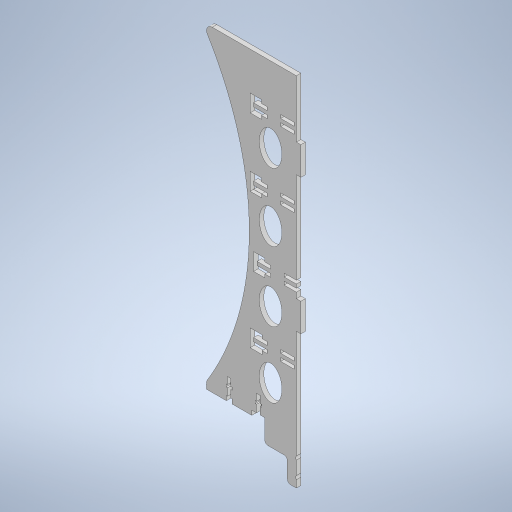
# Autodesk Inventor part: ребро0.5
Saved by Autodesk Inventor 2023.1 (Build 271208000, 208)
## iProperties
Created: 2025-01-17
Part Number: ребро0.5
Material: Типовые
Document SubType Name: Modeling
Designer: Коноваленко
Density: 1 g/cm^3
Appearance: По умолчанию
Author: Коноваленко
Autodesk Inventor part; units mm, degrees
(part 1 of 2)
ref_plane "YZ Plane" through (0, 0, 0) normal (1, 0, 0) x (0, 1, 0)
ref_plane "XZ Plane" through (0, 0, 0) normal (0, 1, 0) x (-1, 0, 0)
ref_plane "XY Plane" through (0, 0, 0) normal (0, 0, 1) x (1, 0, 0)
sketch "Эскиз1" plane through (0, 0, 0) normal (0, 0, 1) x (1, 0, 0)
  line L0 (81.8324, 0) -> (81.8324, -4) construction
  line L1 (72.759, -4) -> (11.9953, -4)
  line L2 (11.9953, -4) -> (11.9953, 0) construction
  line L3 (11.9953, 0) -> (81.8324, 0) construction
  line L4 (-75.5314, 0) -> (7.9958, 0) construction
  line L5 (7.9958, 0) -> (7.9958, -4) construction
  line L6 (7.9958, -4) -> (-66.4579, -4)
  line L7 (-75.5314, -4) -> (-75.5314, 0) construction
  line L8 (7.9953, 276) -> (11.9953, 276) construction
  line L9 (-75.5314, 0) -> (81.8324, 0)
  line L10 (72.759, 276) -> (-66.4579, 276)
  arc A0 (-70.7311, 3.5962) -> (-70.7311, 268.4038) centre (-288.6628, 136) ccw
  line L11 (3.1505, 276) -> (3.1505, 0) construction
  arc A1 (77.0322, 268.4038) -> (77.0322, 3.5962) centre (294.9639, 136) ccw
  arc A2 (-66.4579, 276) -> (-70.7311, 268.4038) centre (-66.4579, 271) ccw
  arc A3 (77.0322, 268.4038) -> (72.759, 276) centre (72.759, 271) ccw
  arc A4 (-70.7311, 3.5962) -> (-66.4579, -4) centre (-66.4579, 1) ccw
  arc A5 (72.759, -4) -> (77.0322, 3.5962) centre (72.759, 1) ccw
  point P0 (81.8324, 276)
  point P1 (-75.5314, 276)
  point P2 (-71.3569, 0)
  point P3 (77.658, 0)
  dimension "d0" = 255
  dimension "d1" = 5
  constraints: 24 end point, 16 point on circle, 8 tangent, 6 centre point, 4 point on line, 3 equal radius, 2 midpoint, 1 horizontal, 1 parallel, 1 symmetric about line, 1 other
  measures "d0" radius of A0
  measures "d1" radius of A2
extrude "Выдавливание1" add sketch "Эскиз1" along normal blind 4
sketch "Эскиз2" plane through (0, 0, 4) normal (0, 0, 1) x (1, 0, 0)
  line L0 (-29.8867, 53.1563) -> (-17.8867, 53.1563)
  line L1 (42.1133, 53.1563) -> (42.1133, 54.9927) construction
  line L2 (-29.8867, 50.1563) -> (-29.8867, 53.1563)
  line L3 (6.1133, 50.1563) -> (6.1133, 53.1563)
  line L4 (6.1133, 50.1563) -> (6.1133, 53.1563) construction
  line L5 (-17.8867, 50.1563) -> (-17.8867, 53.1563)
  line L6 (-5.8867, 50.1563) -> (-5.8867, 53.1563)
  line L7 (18.1133, 50.1563) -> (18.1133, 53.1563)
  line L8 (30.1133, 50.1563) -> (30.1133, 53.1563)
  line L9 (-17.8867, 50.1563) -> (-29.8867, 50.1563)
  line L10 (-17.8867, 53.1563) -> (-5.8867, 53.1563) construction
  line L11 (-5.8867, 53.1563) -> (6.1133, 53.1563)
  line L12 (-5.8867, 50.1563) -> (-17.8867, 50.1563) construction
  line L13 (6.1133, 53.1563) -> (18.1133, 53.1563) construction
  line L14 (18.1133, 50.1563) -> (6.1133, 50.1563) construction
  line L15 (18.1133, 53.1563) -> (30.1133, 53.1563)
  line L16 (30.1133, 53.1563) -> (42.1133, 53.1563) construction
  line L17 (30.1133, 50.1563) -> (18.1133, 50.1563)
  line L18 (6.1133, 50.1563) -> (-5.8867, 50.1563)
  line L19 (6.1133, 6.0367) -> (6.1133, 56.3563) construction
  line L20 (-29.8867, 59.3563) -> (-17.8867, 59.3563)
  line L21 (42.1133, 59.3563) -> (42.1133, 56.3563) construction
  line L22 (42.1133, 56.3563) -> (30.1133, 56.3563) construction
  line L23 (-29.8867, 56.3563) -> (-29.8867, 59.3563)
  line L24 (6.1133, 56.3563) -> (6.1133, 59.3563)
  line L25 (6.1133, 56.3563) -> (6.1133, 59.3563) construction
  line L26 (-17.8867, 56.3563) -> (-17.8867, 59.3563)
  line L27 (-5.8867, 56.3563) -> (-5.8867, 59.3563)
  line L28 (18.1133, 56.3563) -> (18.1133, 59.3563)
  line L29 (30.1133, 56.3563) -> (30.1133, 59.3563)
  line L30 (-17.8867, 56.3563) -> (-29.8867, 56.3563)
  line L31 (-17.8867, 59.3563) -> (-5.8867, 59.3563) construction
  line L32 (-5.8867, 59.3563) -> (6.1133, 59.3563)
  line L33 (-5.8867, 56.3563) -> (-17.8867, 56.3563) construction
  line L34 (6.1133, 59.3563) -> (18.1133, 59.3563) construction
  line L35 (18.1133, 56.3563) -> (6.1133, 56.3563) construction
  line L36 (18.1133, 59.3563) -> (30.1133, 59.3563)
  line L37 (30.1133, 59.3563) -> (42.1133, 59.3563) construction
  line L38 (30.1133, 56.3563) -> (18.1133, 56.3563)
  line L39 (6.1133, 56.3563) -> (-5.8867, 56.3563)
  line L40 (6.1133, -16.2034) -> (6.1133, 259.7966) construction
  line L41 (72.759, 276) -> (-66.4579, 276) projected
  line L42 (9.2728, 110.1563) -> (9.2728, 113.1563)
  line L43 (9.2728, 110.1563) -> (9.2728, 113.1563) construction
  line L44 (-2.8167, 113.1563) -> (9.2728, 113.1563)
  line L45 (9.2728, 110.1563) -> (-2.8167, 110.1563)
  line L46 (-2.8167, 110.1563) -> (-2.8167, 113.1563)
  line L47 (-14.8167, 110.1563) -> (-14.8167, 113.1563)
  line L48 (-14.8167, 113.1563) -> (-2.8167, 113.1563) construction
  line L49 (-2.8167, 110.1563) -> (-14.8167, 110.1563) construction
  line L50 (9.2728, 55.0001) -> (9.2728, 110.1563) construction
  line L51 (21.2728, 110.1563) -> (9.2728, 110.1563) construction
  line L52 (9.2728, 113.1563) -> (21.2728, 113.1563) construction
  line L53 (21.2728, 110.1563) -> (21.2728, 113.1563)
  line L54 (33.2728, 110.1563) -> (21.2728, 110.1563)
  line L55 (21.2728, 113.1563) -> (33.2728, 113.1563)
  line L56 (33.2728, 110.1563) -> (33.2728, 113.1563)
  line L57 (45.1508, 113.1563) -> (45.1508, 110.1563) construction
  line L58 (33.2728, 113.1563) -> (45.1508, 113.1563) construction
  line L59 (-26.8167, 113.1563) -> (-14.8167, 113.1563)
  line L60 (-26.8167, 110.1563) -> (-26.8167, 113.1563)
  line L61 (-14.8167, 110.1563) -> (-26.8167, 110.1563)
  line L62 (-14.8167, 116.3563) -> (-14.8167, 119.3563)
  line L63 (-26.8167, 119.3563) -> (-14.8167, 119.3563)
  line L64 (-14.8167, 116.3563) -> (-26.8167, 116.3563)
  line L65 (21.2728, 116.3563) -> (21.2728, 119.3563)
  line L66 (21.2728, 119.3563) -> (33.2728, 119.3563)
  line L67 (33.2728, 116.3563) -> (33.2728, 119.3563)
  line L68 (33.2728, 116.3563) -> (21.2728, 116.3563)
  line L69 (45.1833, 119.3563) -> (45.1833, 116.3563) construction
  line L70 (21.2728, 116.3563) -> (9.2728, 116.3563) construction
  line L71 (9.2728, 119.3563) -> (21.2728, 119.3563) construction
  line L72 (9.2728, 116.3563) -> (9.2728, 119.3563)
  line L73 (9.2728, 116.3563) -> (9.2728, 119.3563) construction
  line L74 (-26.8167, 116.3563) -> (-26.8167, 119.3563)
  line L75 (33.2728, 119.3563) -> (45.1833, 119.3563) construction
  line L76 (-14.8167, 119.3563) -> (-2.8167, 119.3563) construction
  line L77 (-2.8167, 116.3563) -> (-2.8167, 119.3563)
  line L78 (-2.8167, 119.3563) -> (9.2728, 119.3563)
  line L79 (9.2728, 116.3563) -> (-2.8167, 116.3563)
  line L80 (-2.8167, 116.3563) -> (-14.8167, 116.3563) construction
  line L81 (45.1833, 116.3563) -> (33.2728, 116.3563) construction
  line L82 (6.1133, 170.1563) -> (6.1133, 173.1563)
  line L83 (6.1133, 170.1563) -> (6.1133, 173.1563) construction
  line L84 (-5.8867, 173.1563) -> (6.1133, 173.1563)
  line L85 (6.1133, 170.1563) -> (-5.8867, 170.1563)
  line L86 (-5.8867, 170.1563) -> (-5.8867, 173.1563)
  line L87 (-17.8867, 170.1563) -> (-17.8867, 173.1563)
  line L88 (-17.8867, 173.1563) -> (-5.8867, 173.1563) construction
  line L89 (-5.8867, 170.1563) -> (-17.8867, 170.1563) construction
  line L90 (18.1133, 170.1563) -> (6.1133, 170.1563) construction
  line L91 (6.1133, 173.1563) -> (18.1133, 173.1563) construction
  line L92 (18.1133, 170.1563) -> (18.1133, 173.1563)
  line L93 (30.1133, 170.1563) -> (18.1133, 170.1563)
  line L94 (18.1133, 173.1563) -> (30.1133, 173.1563)
  line L95 (30.1133, 170.1563) -> (30.1133, 173.1563)
  line L96 (42.1133, 170.1563) -> (30.1133, 170.1563) construction
  line L97 (42.1133, 173.1563) -> (42.1133, 170.1563) construction
  line L98 (30.1133, 173.1563) -> (42.1133, 173.1563) construction
  line L99 (-29.8867, 173.1563) -> (-17.8867, 173.1563)
  line L100 (-29.8867, 170.1563) -> (-29.8867, 173.1563)
  line L101 (-17.8867, 170.1563) -> (-29.8867, 170.1563)
  line L102 (6.1133, 179.3563) -> (18.1133, 179.3563) construction
  line L103 (18.1133, 176.3563) -> (6.1133, 176.3563) construction
  line L104 (18.1133, 176.3563) -> (18.1133, 179.3563)
  line L105 (30.1133, 176.3563) -> (18.1133, 176.3563)
  line L106 (18.1133, 179.3563) -> (30.1133, 179.3563)
  line L107 (-29.8867, 179.3563) -> (-17.8867, 179.3563)
  line L108 (-17.8867, 176.3563) -> (-29.8867, 176.3563)
  line L109 (-29.8867, 176.3563) -> (-29.8867, 179.3563)
  line L110 (-17.8867, 176.3563) -> (-17.8867, 179.3563)
  line L111 (30.1133, 176.3563) -> (30.1133, 179.3563)
  line L112 (42.1133, 176.3563) -> (30.1133, 176.3563) construction
  line L113 (42.1133, 179.3563) -> (42.1133, 176.3563) construction
  line L114 (30.1133, 179.3563) -> (42.1133, 179.3563) construction
  line L115 (-5.8867, 176.3563) -> (-17.8867, 176.3563) construction
  line L116 (-17.8867, 179.3563) -> (-5.8867, 179.3563) construction
  line L117 (-5.8867, 176.3563) -> (-5.8867, 179.3563)
  line L118 (6.1133, 176.3563) -> (-5.8867, 176.3563)
  line L119 (-5.8867, 179.3563) -> (6.1133, 179.3563)
  line L120 (6.1133, 176.3563) -> (6.1133, 179.3563)
  line L121 (6.1133, 176.3563) -> (6.1133, 179.3563) construction
  line L122 (6.1133, 233.1563) -> (18.1133, 233.1563) construction
  line L123 (18.1133, 230.1563) -> (6.1133, 230.1563) construction
  line L124 (18.1133, 230.1563) -> (18.1133, 233.1563)
  line L125 (30.1133, 230.1563) -> (18.1133, 230.1563)
  line L126 (18.1133, 233.1563) -> (30.1133, 233.1563)
  line L127 (-29.8867, 233.1563) -> (-17.8867, 233.1563)
  line L128 (-17.8867, 230.1563) -> (-29.8867, 230.1563)
  line L129 (-29.8867, 230.1563) -> (-29.8867, 233.1563)
  line L130 (-17.8867, 230.1563) -> (-17.8867, 233.1563)
  line L131 (30.1133, 230.1563) -> (30.1133, 233.1563)
  line L132 (42.1133, 230.1563) -> (30.1133, 230.1563) construction
  line L133 (42.1133, 233.1563) -> (42.1133, 230.1563) construction
  line L134 (30.1133, 233.1563) -> (42.1133, 233.1563) construction
  line L135 (-5.8867, 230.1563) -> (-17.8867, 230.1563) construction
  line L136 (-17.8867, 233.1563) -> (-5.8867, 233.1563) construction
  line L137 (-5.8867, 230.1563) -> (-5.8867, 233.1563)
  line L138 (6.1133, 230.1563) -> (-5.8867, 230.1563)
  line L139 (-5.8867, 233.1563) -> (6.1133, 233.1563)
  line L140 (6.1133, 230.1563) -> (6.1133, 233.1563)
  line L141 (6.1133, 230.1563) -> (6.1133, 233.1563) construction
  line L142 (18.1133, 236.3563) -> (18.1133, 239.3563)
  line L143 (30.1133, 236.3563) -> (18.1133, 236.3563)
  line L144 (18.1133, 239.3563) -> (30.1133, 239.3563)
  line L145 (30.1133, 236.3563) -> (30.1133, 239.3563)
  line L146 (42.1133, 236.3563) -> (30.1133, 236.3563) construction
  line L147 (30.1133, 239.3563) -> (42.1133, 239.3563) construction
  line L148 (42.1133, 239.3563) -> (42.1133, 236.3563) construction
  line L149 (18.1133, 236.3563) -> (6.1133, 236.3563) construction
  line L150 (6.1133, 239.3563) -> (18.1133, 239.3563) construction
  line L151 (6.1133, 236.3563) -> (6.1133, 239.3563)
  line L152 (6.1133, 236.3563) -> (6.1133, 239.3563) construction
  line L153 (6.1133, 236.3563) -> (-5.8867, 236.3563)
  line L154 (-5.8867, 239.3563) -> (6.1133, 239.3563)
  line L155 (-5.8867, 236.3563) -> (-5.8867, 239.3563)
  line L156 (-5.8867, 236.3563) -> (-17.8867, 236.3563) construction
  line L157 (-17.8867, 239.3563) -> (-5.8867, 239.3563) construction
  line L158 (-17.8867, 236.3563) -> (-17.8867, 239.3563)
  line L159 (-29.8867, 239.3563) -> (-17.8867, 239.3563)
  line L160 (-29.8867, 236.3563) -> (-29.8867, 239.3563)
  line L161 (-17.8867, 236.3563) -> (-29.8867, 236.3563)
  arc A0 (-70.7311, 3.5962) -> (-70.7311, 268.4038) centre (-288.6628, 136) ccw construction
  arc A1 (77.0322, 268.4038) -> (77.0322, 3.5962) centre (294.9639, 136) ccw construction
  line L162 (11.994, 50.1563) -> (7.994, 50.1563) projected
  line L163 (11.994, 110.1563) -> (7.994, 110.1563) projected
  line L164 (11.9939, 170.1563) -> (7.9939, 170.1563) projected
  line L165 (11.9939, 230.1563) -> (7.9939, 230.1563) projected
  point P0 (0, 0)
  point P1 (-29.8867, 51.6563)
  point P2 (-17.8867, 51.6563)
  point P3 (-5.8867, 51.6563)
  point P4 (6.1133, 51.6563)
  point P5 (18.1133, 51.6563)
  point P6 (30.1133, 51.6563)
  point P7 (6.1133, 57.8563)
  point P8 (-29.8867, 57.8563)
  point P9 (-17.8867, 57.8563)
  point P10 (-5.8867, 57.8563)
  point P11 (6.1133, 57.8563)
  point P12 (18.1133, 57.8563)
  point P13 (30.1133, 57.8563)
  point P14 (6.1133, 117.4846)
  point P15 (9.2638, 118.9846)
  point P16 (9.2728, 111.6563)
  point P17 (-2.8167, 111.6563)
  point P18 (21.2728, 111.6563)
  point P19 (33.2728, 111.6563)
  point P20 (-14.8167, 111.6563)
  point P21 (-26.8167, 111.6563)
  point P22 (6.1133, 123.6846)
  point P23 (6.1133, 123.6846)
  point P24 (21.2728, 117.8563)
  point P25 (33.2728, 117.8563)
  point P26 (9.2728, 117.8563)
  point P27 (-26.8167, 117.8563)
  point P28 (-2.8167, 117.8563)
  point P29 (-14.8167, 117.8563)
  point P30 (9.2638, 125.1846)
  point P31 (3.228, 119.3563)
  point P32 (30.1133, 171.6563)
  point P33 (-17.8867, 171.6563)
  point P34 (-29.8867, 171.6563)
  point P35 (6.1133, 177.1846)
  point P36 (-17.8867, 177.8563)
  point P37 (-29.8867, 177.8563)
  point P38 (30.1133, 177.8563)
  point P39 (6.1133, 177.8563)
  point P40 (6.1133, 225.9846)
  point P41 (6.1133, 225.9846)
  point P42 (18.1133, 231.6563)
  point P43 (-17.8867, 231.6563)
  point P44 (-29.8867, 231.6563)
  point P45 (30.1133, 231.6563)
  point P46 (-5.8867, 231.6563)
  point P47 (18.1133, 237.8563)
  point P48 (30.1133, 237.8563)
  point P49 (-5.8867, 237.8563)
  point P50 (-17.8867, 237.8563)
  point P51 (-29.8867, 237.8563)
  point P52 (6.1133, 232.1846)
  point P53 (6.1133, 225.1563)
  point P54 (0.1133, 179.3563)
  point P55 (9.994, 50.1563)
  point P56 (9.994, 110.1563)
  point P57 (9.9939, 170.1563)
  point P58 (9.9939, 230.1563)
  dimension "d18" = 12
  dimension "d19" = 12
  dimension "d20" = 12
  dimension "d21" = 12
  dimension "d22" = 4.7
  dimension "d23" = 72
  dimension "d25" = 12
  dimension "d26" = 12
  dimension "d27" = 12
  dimension "d28" = 12
  dimension "d39" = 12
  dimension "d40" = 12
  dimension "d41" = 12
  dimension "d42" = 12
  dimension "d44" = 72
  dimension "d46" = 12
  dimension "d47" = 12
  dimension "d48" = 12
  dimension "d49" = 12
  dimension "d54" = 12
  dimension "d59" = 72
  dimension "d60" = 3
  dimension "d61" = 12
  dimension "d66" = 72
  dimension "d68" = 12
  dimension "d69" = 12
  dimension "d71" = 12
  dimension "d74" = 3
  dimension "d75" = 12
  dimension "d76" = 12
  dimension "d78" = 12
  dimension "d79" = 45.8
  dimension "d97" = 3.2
  dimension "d98" = 3
  dimension "d99" = 3.2
  dimension "d100" = 3
  dimension "d101" = 3.2
  dimension "d102" = 3.2
  constraints: 322 end point, 284 parallel, 238 perpendicular, 91 point on line, 48 horizontal, 47 midpoint, 11 vertical, 8 equal length
  measures "d18" distance of point (-29.887, 51.656) point (-17.887, 51.656)
  measures "d19" distance of point (-5.887, 51.656) point (-17.887, 51.656)
  measures "d20" distance of point (6.113, 51.656) point (18.113, 51.656)
  measures "d21" distance of point (30.113, 51.656) point (18.113, 51.656)
  measures "d22" distance from line of point (6.113, 57.856) L11
  measures "d23" distance of L22.start L23.start
  measures "d25" distance of point (-29.887, 57.856) point (-17.887, 57.856)
  measures "d26" distance of point (-5.887, 57.856) point (-17.887, 57.856)
  measures "d27" distance of point (6.113, 57.856) point (18.113, 57.856)
  measures "d28" distance of point (30.113, 57.856) point (18.113, 57.856)
  measures "d39" distance of point (-26.817, 111.656) point (-14.817, 111.656)
  measures "d40" distance of point (-2.817, 111.656) point (-14.817, 111.656)
  measures "d41" distance of point (9.273, 111.656) point (21.273, 111.656)
  measures "d42" distance of point (33.273, 111.656) point (21.273, 111.656)
  measures "d44" distance of L81.start L64.end
  measures "d46" distance of point (-26.817, 117.856) point (-14.817, 117.856)
  measures "d47" distance of point (-2.817, 117.856) point (-14.817, 117.856)
  measures "d48" distance of point (9.273, 117.856) point (21.273, 117.856)
  measures "d49" distance of point (33.273, 117.856) point (21.273, 117.856)
  measures "d54" distance of point (-29.887, 171.656) point (-17.887, 171.656)
  measures "d59" distance of L112.start L109.start
  measures "d60" distance of L114.end L112.start
  measures "d61" distance of point (-29.887, 177.856) point (-17.887, 177.856)
  measures "d66" distance of L132.start L128.end
  measures "d68" distance of point (-29.887, 231.656) point (-17.887, 231.656)
  measures "d69" distance of point (-5.887, 231.656) point (-17.887, 231.656)
  measures "d71" distance of point (30.113, 231.656) point (18.113, 231.656)
  measures "d74" distance of L147.end L146.start
  measures "d75" distance of point (-29.887, 237.856) point (-17.887, 237.856)
  measures "d76" distance of point (-5.887, 237.856) point (-17.887, 237.856)
  measures "d78" distance of point (30.113, 237.856) point (18.113, 237.856)
  measures "d79" vertical distance of point (6.113, 225.156) point (0.113, 179.356)
  measures "d97" distance of L0.start L23.start
  measures "d98" distance of L8.start L8.end
  measures "d99" distance between parallel lines of L55 L68
  measures "d100" distance of L61.end L59.start
  measures "d101" distance between parallel lines of L94 L105
  measures "d102" distance between parallel lines of L126 L143
extrude "Выдавливание2" cut sketch "Эскиз2" against normal blind 10
sketch "Эскиз3" plane through (0, 0, 0) normal (0, 0, -1) x (-1, 0, 0)
  line L0 (29.8867, 239.3563) -> (29.8867, 236.3563)
  line L1 (5.8867, 236.3563) -> (5.8867, 239.3563) construction
  line L2 (29.8867, 239.3563) -> (17.8867, 239.3563) construction
  line L3 (5.8867, 239.3563) -> (17.8867, 239.3563) construction
  line L4 (17.8867, 239.3563) -> (17.8867, 287.0573) construction
  line L5 (-72.759, 276) -> (66.4579, 276) construction
  line L6 (-72.759, 276) -> (66.4579, 276) projected
  line L7 (-3.1505, 276) -> (-3.1505, 0) construction
  ellipse E0 centre (14.8167, 209.3563) end of major axis (14.8167, 194.3563) minor radius 10
  ellipse E1 centre (14.8167, 149.3563) end of major axis (14.8167, 134.3563) minor radius 10
  line L8 (26.9717, 119.3563) -> (14.9717, 119.3563) construction
  line L9 (14.9717, 119.3563) -> (26.9717, 119.3563)
  ellipse E2 centre (-30.1133, 259.231) end of major axis (-46.1133, 259.231) minor radius 10
  line L10 (-30.1133, 236.3563) -> (-30.1133, 239.3563) projected
  line L11 (-18.1133, 239.3563) -> (-30.1133, 239.3563) projected
  line L12 (-30.1133, 239.3563) -> (-30.1133, 283.7222) construction
  line L13 (26.8167, 119.3563) -> (14.8167, 119.3563) projected
  line L14 (14.8167, 119.3563) -> (14.8167, 279.8353) construction
  line L15 (14.8167, 119.3563) -> (175.2957, 119.3563) construction
  line L16 (14.8167, 119.3563) -> (14.8167, -15.3407) construction
  ellipse E3 centre (14.8167, 87.8563) end of major axis (14.8167, 72.8563) minor radius 10
  ellipse E4 centre (14.8167, 29.3563) end of major axis (14.8167, 14.3563) minor radius 10
  line L17 (14.8167, 116.3563) -> (14.8167, 119.3563) projected
  point P0 (0, 0)
  point P1 (-33.2728, 119.3563)
  point P2 (-21.2728, 119.3563)
  point P3 (17.8867, 179.3563)
  point P4 (17.8867, 59.3563)
  point P5 (14.8167, 117.8563)
  dimension "d92" = 16
  dimension "d90" = 160.479
  dimension "d91" = 90
  dimension "d93" = 30
  dimension "d94" = 30
  dimension "d95" = 30
  dimension "d96" = 30
  constraints: 20 end point, 5 point on line, 4 centre point, 3 perpendicular, 3 vertical, 2 horizontal, 2 midpoint, 2 symmetric about line, 2 other
  measures "d90" distance of L13.end L14.end
  measures "d91" angle of L15 L14
  measures "d93" vertical distance of L2.end E0.centre
  measures "d94" vertical distance of E1.centre point (17.887, 179.356)
  measures "d95" distance of E3.centre point (14.817, 117.856)
  measures "d96" vertical distance of E4.centre point (17.887, 59.356)
extrude "Выдавливание3" cut sketch "Эскиз3" against normal blind 10
sketch "Эскиз4" plane through (-71.3569, 0, 0) normal (0, -1, 0) x (1, 0, 0)
  line L0 (91.3569, 4) -> (51.3569, 4)
  line L1 (51.3569, 4) -> (51.3569, 0)
  line L2 (51.3569, 0) -> (91.3569, 0)
  line L3 (91.3569, 0) -> (91.3569, 4)
  line L4 (72.8558, 3.5003) -> (72.8557, 3.5003) projected
  point P0 (71.3569, 0)
  point P1 (0, 4)
  point P2 (149.0149, 4)
  dimension "d103" = 40
  dimension "d104" = 4
  constraints: 8 end point, 2 parallel, 1 horizontal, 1 midpoint, 1 perpendicular
  measures "d103" distance of L1.end L2.end
  measures "d104" distance of L0.end L1.end
extrude "Выдавливание4" add sketch "Эскиз4" along normal blind 20
sketch "Эскиз5" plane through (0, 0, 0) normal (0, 0, -1) x (-1, 0, 0)
  line L0 (0, -20) -> (-20, -20)
  line L1 (-20, -20) -> (-20, -40)
  line L2 (-20, -40) -> (0, -40)
  line L3 (0, -40) -> (0, -20)
  line L4 (20, -20) -> (-20, -20) projected
  point P0 (0, 0)
  point P1 (17, -20)
  point P2 (-17, -20)
  point P3 (0, -20)
  dimension "d108" = 20
  dimension "d109" = 20
  constraints: 8 end point, 2 parallel, 1 horizontal, 1 midpoint, 1 perpendicular
  measures "d108" distance of L2.end L1.end
  measures "d109" distance of L0.end L1.end
extrude "Выдавливание5" add sketch "Эскиз5" against normal blind 4
fillet "Сопряжение2" radius 3 3 edges at (20, -40, 2) (0, -40, 2) (0, -20, 2)
fillet "Сопряжение3" radius 3 1 edges at (-20, -20, 2)
sketch "Эскиз6" plane through (0, 0, 0) normal (0, 0, -1) x (-1, 0, 0)
  line L0 (0, -37) -> (0, -23) projected
  line L1 (-20, 0) -> (-20, -37) projected
  line L2 (0, -23) -> (0, -37) projected
  circle A0 centre (-10, -32) radius 2.55
  circle A1 centre (-10, -17) radius 2.55
  line L3 (-10, -17) -> (-10, -32) construction
  line L4 (-17, -40) -> (-3, -40) projected
  line L5 (-10, -32) -> (-20, -32) construction
  line L6 (-10, -32) -> (0, -32) construction
  point P0 (0, 0)
  point P1 (-10, -40)
  dimension "d121" = 5.1
  dimension "d122" = 5.1
  dimension "d123" = 8
  dimension "d124" = 15
  constraints: 6 end point, 3 point on line, 2 centre point, 1 collinear, 1 midpoint, 1 parallel, 1 perpendicular
  measures "d121" diameter of A1
  measures "d122" diameter of A0
  measures "d123" distance of point (-10, -40) L3.end
  measures "d124" distance of L3.start L3.end
extrude "Выдавливание6" cut sketch "Эскиз6" against normal blind 4
sketch "Эскиз7" plane through (0, 0, 0) normal (0, 0, -1) x (-1, 0, 0)
  circle A0 centre (-38.6107, 23.1063) radius 10
  point P0 (0, 0)
  dimension "d125" = 20
  constraints: 1 centre point
  measures "d125" diameter of A0
extrude "Выдавливание7" cut sketch "Эскиз7" against normal blind 4
sketch "Эскиз8" plane through (77.658, 0, 0) normal (0, -1, 0) x (1, 0, 0)
  line L0 (-57.658, 4) -> (0, 4) construction
  line L1 (-57.658, 0) -> (0, 0) construction
  line L2 (0, 4) -> (-17.5, 4)
  line L3 (-17.5, 4) -> (-17.5, 0)
  line L4 (-17.5, 0) -> (0, 0)
  line L5 (0, 0) -> (0, 4)
  line L6 (-22.5, 4) -> (-40, 4)
  line L7 (-40, 4) -> (-40, 0)
  line L8 (-40, 0) -> (-22.5, 0)
  line L9 (-22.5, 0) -> (-22.5, 4)
  line L10 (-148.3891, 0) -> (-149.1159, 0) projected
  line L11 (-149.0149, 4) -> (-97.658, 4) projected
  line L12 (-149.1159, 0) -> (-131.6159, 0)
  line L13 (-131.6159, 0) -> (-131.6159, 4)
  line L14 (-131.6159, 4) -> (-149.1159, 4)
  line L15 (-149.1159, 4) -> (-149.1159, 0)
  line L16 (-149.0149, 0) -> (-97.658, 0) projected
  line L17 (-126.6159, 0) -> (-109.1159, 0)
  line L18 (-109.1159, 0) -> (-109.1159, 4)
  line L19 (-109.1159, 4) -> (-126.6159, 4)
  line L20 (-126.6159, 4) -> (-126.6159, 0)
  point P0 (-77.658, 0)
  point P1 (-17.5, 4)
  point P2 (-131.6159, 2)
  point P3 (-126.6159, 2)
  point P4 (-126.6159, 4)
  dimension "d128" = 17.5
  dimension "d137" = 17.5
  dimension "d138" = 5
  dimension "d139" = 17.5
  dimension "d140" = 17.5
  dimension "d141" = 5
  constraints: 32 end point, 8 parallel, 6 point on line, 4 horizontal, 4 perpendicular, 2 midpoint
  measures "d128" distance of L4.end L3.end
  measures "d137" distance of L6.start L6.end
  measures "d138" distance between parallel lines of L9 L3
  measures "d139" distance of L14.end L13.end
  measures "d140" distance of L19.end L18.end
  measures "d141" distance of point (-131.616, 2) point (-126.616, 2)
extrude "Выдавливание8" add sketch "Эскиз8" along normal blind 4 contours L5 L4 L3 L2 | L9 L8 L7 L6 | L10 L15 L14 L11 L13 L12 | L20 L11 L18 L16
sketch "Эскиз9" plane through (0, 0, 4) normal (0, 0, 1) x (1, 0, 0)
  line L0 (-27.304, 0) -> (-24.154, 0)
  line L1 (-24.154, 15) -> (-27.304, 15)
  line L2 (-22.979, 8.8) -> (-22.979, 6.5)
  line L3 (-28.479, 6.5) -> (-28.479, 8.8)
  line L4 (-25.729, 15) -> (-25.729, 0) construction
  line L5 (-28.479, 8.8) -> (-27.304, 8.8)
  line L6 (-24.154, 8.8) -> (-22.979, 8.8)
  line L7 (-27.304, 15) -> (-27.304, 8.8)
  line L8 (-27.304, 6.5) -> (-27.304, 0)
  line L9 (-22.979, 6.5) -> (-24.154, 6.5)
  line L10 (-27.304, 6.5) -> (-28.479, 6.5)
  line L11 (-24.154, 0) -> (-24.154, 6.5)
  line L12 (-24.154, 8.8) -> (-24.154, 15)
  line L13 (-52.8263, 0) -> (-50.0896, 0)
  line L14 (-49.8829, 14.9986) -> (-53.0329, 14.9986)
  line L15 (-48.7079, 8.8) -> (-48.7079, 6.5)
  line L16 (-54.2079, 6.5) -> (-54.2079, 8.8)
  line L17 (-51.4579, 14.9986) -> (-51.4579, 0) construction
  line L18 (-54.2079, 8.8) -> (-53.0329, 8.8)
  line L19 (-49.8829, 8.8) -> (-48.7079, 8.8)
  line L20 (-53.0329, 14.9986) -> (-53.0329, 8.8)
  line L21 (-52.8263, 6.5) -> (-52.8263, 0)
  line L22 (-48.7079, 6.5) -> (-50.0896, 6.5)
  line L23 (-52.8263, 6.5) -> (-54.2079, 6.5)
  line L24 (-50.0896, 0) -> (-50.0896, 6.5)
  line L25 (-49.8829, 8.8) -> (-49.8829, 14.9986)
  line L26 (-53.9579, 0) -> (-48.9579, 0) projected
  line L27 (-52.8263, 6.5) -> (-50.0896, 6.5) construction
  line L28 (30.404, 0) -> (27.254, 0)
  line L29 (27.254, 15) -> (30.404, 15)
  line L30 (20, 0) -> (37.658, 0) projected
  line L31 (26.079, 6.5) -> (26.079, 8.8)
  line L32 (31.579, 8.8) -> (31.579, 6.5)
  line L33 (28.829, 15) -> (28.829, 0) construction
  line L34 (26.079, 8.8) -> (27.254, 8.8)
  line L35 (30.404, 8.8) -> (31.579, 8.8)
  line L36 (27.254, 0) -> (27.254, 6.5)
  line L37 (27.254, 8.8) -> (27.254, 15)
  line L38 (30.404, 15) -> (30.404, 8.8)
  line L39 (30.404, 6.5) -> (30.404, 0)
  line L40 (31.579, 6.5) -> (30.404, 6.5)
  line L41 (27.254, 6.5) -> (26.079, 6.5)
  line L42 (59.233, 0) -> (56.083, 0)
  line L43 (56.083, 15) -> (59.233, 15)
  line L44 (60.408, 6.5) -> (60.408, 8.8)
  line L45 (54.908, 8.8) -> (54.908, 6.5)
  line L46 (55.158, 0) -> (60.158, 0) projected
  line L47 (57.658, 15) -> (57.658, 0) construction
  line L48 (60.408, 8.8) -> (59.233, 8.8)
  line L49 (56.083, 8.8) -> (54.908, 8.8)
  line L50 (56.083, 0) -> (56.083, 6.5)
  line L51 (56.083, 8.8) -> (56.083, 15)
  line L52 (54.908, 6.5) -> (56.083, 6.5)
  line L53 (59.233, 6.5) -> (60.408, 6.5)
  line L54 (59.233, 15) -> (59.233, 8.8)
  line L55 (59.233, 6.5) -> (59.233, 0)
  point P0 (0, 0)
  point P1 (-31.4579, 0)
  point P2 (-49.3988, 6.5)
  dimension "d132" = 15
  dimension "d133" = 3.15
  dimension "d134" = 2.3
  dimension "d135" = 5.5
  dimension "d142" = 15
  dimension "d143" = 3.15
  dimension "d144" = 2.3
  dimension "d145" = 5.5
  dimension "d146" = 6.5
  dimension "d154" = 3.15
  dimension "d155" = 15
  dimension "d156" = 5.5
  dimension "d157" = 2.3
  dimension "d159" = 3.15
  dimension "d160" = 15
  dimension "d161" = 5.5
  dimension "d162" = 2.3
  constraints: 106 end point, 40 parallel, 16 perpendicular, 13 horizontal, 12 midpoint, 5 equal length, 4 vertical
  measures "d132" distance of L0.end L1.start
  measures "d133" distance of L1.start L1.end
  measures "d134" distance of L2.start L2.end
  measures "d135" distance of L3.end L2.start
  measures "d142" distance of L24.start L25.end
  measures "d143" distance of L25.end L14.end
  measures "d144" distance of L15.start L15.end
  measures "d145" distance of L16.end L15.start
  measures "d146" vertical distance of L24.start point (-49.399, 6.5)
  measures "d154" distance of L29.start L29.end
  measures "d155" distance of L28.end L29.start
  measures "d156" distance of L31.end L32.start
  measures "d157" distance of L31.start L31.end
  measures "d159" distance of L43.start L43.end
  measures "d160" distance of L42.end L43.start
  measures "d161" distance of L45.start L44.end
  measures "d162" distance of L44.end L44.start
extrude "Выдавливание9" cut sketch "Эскиз9" against normal blind 4
sketch "Эскиз13" plane through (0, 0, 0) normal (0, 0, -1) x (-1, 0, 0)
  line L0 (-7.9955, 45.1563) -> (-11.9955, 45.1563) construction
  line L1 (-11.9955, 45.1563) -> (-11.9955, 80.1563) construction
  line L2 (-11.9955, 80.1563) -> (-7.9955, 80.1563) construction
  line L3 (-7.9955, 80.1563) -> (-7.9955, 45.1563) construction
  line L4 (-11.9955, 140.1563) -> (-7.9955, 140.1563) construction
  line L5 (-7.9955, 140.1563) -> (-7.9955, 105.1563) construction
  line L6 (-7.9955, 105.1563) -> (-11.9955, 105.1563) construction
  line L7 (-11.9955, 105.1563) -> (-11.9955, 140.1563) construction
  line L8 (-7.9955, 165.1563) -> (-11.9955, 165.1563) construction
  line L9 (-11.9955, 165.1563) -> (-11.9955, 200.1563) construction
  line L10 (-11.9955, 200.1563) -> (-7.9955, 200.1563) construction
  line L11 (-7.9955, 200.1563) -> (-7.9955, 165.1563) construction
  line L12 (-11.9955, 256) -> (-7.9955, 256) construction
  line L13 (-7.9955, 256) -> (-7.9955, 225.1563) construction
  line L14 (-7.9955, 225.1563) -> (-11.9955, 225.1563) construction
  line L15 (-11.9955, 225.1563) -> (-11.9955, 256) construction
  line L16 (-11.9955, 80.1563) -> (-7.9955, 80.1563)
  arc A0 (-77.0322, 3.5962) -> (-77.658, 0) centre (-72.759, 1) ccw projected
  arc A1 (-77.0322, 3.5962) -> (-77.0322, 268.4038) centre (-294.9639, 136) ccw projected
  arc A2 (-72.759, 276) -> (-77.0322, 268.4038) centre (-72.759, 271) ccw projected
  line L17 (-77.658, 0) -> (-77.658, -50.632)
  line L18 (-11.9955, -50.632) -> (-77.658, -50.632)
  line L19 (-7.9955, 0) -> (-11.9955, 0)
  line L20 (-7.9955, 0) -> (-7.9955, -50.632)
  line L21 (-7.9955, -50.632) -> (-11.9955, -50.632)
  line L22 (-7.9955, 256) -> (-7.9955, 276)
  line L23 (-72.759, 276) -> (-7.9955, 276)
  line L24 (-72.759, 276) -> (66.4579, 276) projected
  line L25 (-7.9955, 256) -> (-7.9955, 225.1563)
  line L26 (-7.9955, 165.1563) -> (-7.9955, 140.1563)
  line L27 (-7.9955, 225.1563) -> (-11.9955, 225.1563)
  line L28 (-11.9955, 225.1563) -> (-11.9955, 200.1563)
  line L29 (-11.9955, 200.1563) -> (-7.9955, 200.1563)
  line L30 (-7.9955, 200.1563) -> (-7.9955, 165.1563)
  line L31 (-7.9955, 140.1563) -> (-7.9955, 105.1563)
  line L32 (-7.9955, 105.1563) -> (-11.9955, 105.1563)
  line L33 (-11.9955, 105.1563) -> (-11.9955, 80.1563)
  line L34 (-7.9955, 80.1563) -> (-7.9955, 0)
  point P0 (0, 0)
  constraints: 68 end point, 5 perpendicular, 4 collinear, 4 vertical, 32 other
extrude "Выдавливание11" cut sketch "Эскиз13" against normal blind 10
sketch "Эскиз14" plane through (0, 0, 0) normal (0, 0, -1) x (-1, 0, 0)
  line L0 (-6.5205, -8.0916) -> (22.4522, -8.0916) construction
  line L1 (22.4522, -8.0916) -> (22.4522, -20.3744) construction
  line L2 (22.4522, -20.3744) -> (-6.5205, -20.3744) construction
  line L3 (-6.5205, -20.3744) -> (-6.5205, -8.0916) construction
  line L4 (-5.5687, -9.3874) -> (-5.5687, -10.7429)
  spline S0 degree 2 poles (-5.5687, -10.7429) (-5.5687, -11.0295) (-5.5064, -11.1042) knots 0 0 0 1 1 1
  spline S1 degree 2 poles (-5.5064, -11.1042) (-5.4216, -11.2039) (-5.2821, -11.2039) knots 0 0 0 1 1 1
  line L5 (-5.2821, -11.2039) -> (-5.0952, -11.2039)
  line L6 (-5.0952, -11.2039) -> (-5.0952, -11.2861)
  line L7 (-5.0952, -11.2861) -> (-6.3287, -11.2861)
  line L8 (-6.3287, -11.2861) -> (-6.3287, -11.2039)
  line L9 (-6.3287, -11.2039) -> (-6.2365, -11.2039)
  spline S2 degree 2 poles (-6.2365, -11.2039) (-6.1468, -11.2039) (-5.9998, -11.1142) (-5.9424, -10.9622) (-5.9424, -10.7429) knots 0 0 0 1 2 3 3 3
  line L10 (-5.9424, -10.7429) -> (-5.9424, -9.3874)
  line L11 (-5.9424, -9.3874) -> (-6.3436, -9.3874)
  line L12 (-6.3436, -9.3874) -> (-6.3436, -9.2254)
  line L13 (-6.3436, -9.2254) -> (-5.9424, -9.2254)
  line L14 (-5.9424, -9.2254) -> (-5.9424, -9.0908)
  spline S3 degree 2 poles (-5.9424, -9.0908) (-5.9424, -8.7818) (-5.7431, -8.3557) (-5.3344, -8.0916) (-5.0803, -8.0916) knots 0 0 0 1 2 3 3 3
  spline S4 degree 2 poles (-5.0803, -8.0916) (-4.8435, -8.0916) (-4.6442, -8.2436) knots 0 0 0 1 1 1
  spline S5 degree 2 poles (-4.6442, -8.2436) (-4.5146, -8.3458) (-4.5146, -8.4704) knots 0 0 0 1 1 1
  spline S6 degree 2 poles (-4.5146, -8.4704) (-4.5146, -8.5376) (-4.6317, -8.6572) (-4.699, -8.6572) knots 0 0 0 1 2 2 2
  spline S7 degree 2 poles (-4.699, -8.6572) (-4.7513, -8.6572) (-4.866, -8.5825) (-5.0329, -8.3383) (-5.1027, -8.2959) knots 0 0 0 1 2 3 3 3
  spline S8 degree 2 poles (-5.1027, -8.2959) (-5.1725, -8.2536) (-5.2572, -8.2536) knots 0 0 0 1 1 1
  spline S9 degree 2 poles (-5.2572, -8.2536) (-5.3618, -8.2536) (-5.5064, -8.3632) (-5.5687, -8.595) (-5.5687, -9.0759) knots 0 0 0 1 2 3 3 3
  line L15 (-5.5687, -9.0759) -> (-5.5687, -9.2254)
  line L16 (-5.5687, -9.2254) -> (-5.0379, -9.2254)
  line L17 (-5.0379, -9.2254) -> (-5.0379, -9.3874)
  line L18 (-5.0379, -9.3874) -> (-5.5687, -9.3874)
  line L19 (-4.2355, -9.1656) -> (-4.2355, -9.6291)
  spline S10 degree 2 poles (-4.2355, -9.6291) (-3.9764, -9.1656) (-3.7048, -9.1656) knots 0 0 0 1 1 1
  spline S11 degree 2 poles (-3.7048, -9.1656) (-3.5827, -9.1656) (-3.4207, -9.3151) (-3.4207, -9.4148) knots 0 0 0 1 2 2 2
  spline S12 degree 2 poles (-3.4207, -9.4148) (-3.4207, -9.502) (-3.5378, -9.6241) (-3.6176, -9.6241) knots 0 0 0 1 2 2 2
  spline S13 degree 2 poles (-3.6176, -9.6241) (-3.6973, -9.6241) (-3.8917, -9.4696) (-3.939, -9.4696) knots 0 0 0 1 2 2 2
  spline S14 degree 2 poles (-3.939, -9.4696) (-3.9789, -9.4696) (-4.0262, -9.5144) knots 0 0 0 1 1 1
  spline S15 degree 2 poles (-4.0262, -9.5144) (-4.1284, -9.6066) (-4.2355, -9.8184) knots 0 0 0 1 1 1
  line L20 (-4.2355, -9.8184) -> (-4.2355, -10.8052)
  spline S16 degree 2 poles (-4.2355, -10.8052) (-4.2355, -10.9771) (-4.1932, -11.0644) knots 0 0 0 1 1 1
  spline S17 degree 2 poles (-4.1932, -11.0644) (-4.1633, -11.1242) (-4.0163, -11.2039) (-3.8767, -11.2039) knots 0 0 0 1 2 2 2
  line L21 (-3.8767, -11.2039) -> (-3.8767, -11.2861)
  line L22 (-3.8767, -11.2861) -> (-4.9332, -11.2861)
  line L23 (-4.9332, -11.2861) -> (-4.9332, -11.2039)
  spline S18 degree 2 poles (-4.9332, -11.2039) (-4.7763, -11.2039) (-4.699, -11.1541) knots 0 0 0 1 1 1
  spline S19 degree 2 poles (-4.699, -11.1541) (-4.6442, -11.1192) (-4.6218, -11.0394) knots 0 0 0 1 1 1
  spline S20 degree 2 poles (-4.6218, -11.0394) (-4.6093, -10.9996) (-4.6093, -10.8202) knots 0 0 0 1 1 1
  line L24 (-4.6093, -10.8202) -> (-4.6093, -10.0253)
  spline S21 degree 2 poles (-4.6093, -10.0253) (-4.6093, -9.6664) (-4.6392, -9.5294) (-4.7165, -9.4646) (-4.7763, -9.4646) knots 0 0 0 1 2 3 3 3
  spline S22 degree 2 poles (-4.7763, -9.4646) (-4.846, -9.4646) (-4.9332, -9.4995) knots 0 0 0 1 1 1
  line L25 (-4.9332, -9.4995) -> (-4.9557, -9.4173)
  line L26 (-4.9557, -9.4173) -> (-4.3302, -9.1656)
  line L27 (-4.3302, -9.1656) -> (-4.2355, -9.1656)
  spline S23 degree 2 poles (-2.2994, -9.1656) (-1.8309, -9.1656) (-1.5493, -9.5219) knots 0 0 0 1 1 1
  spline S24 degree 2 poles (-1.5493, -9.5219) (-1.3076, -9.8234) (-1.3076, -10.2171) knots 0 0 0 1 1 1
  spline S25 degree 2 poles (-1.3076, -10.2171) (-1.3076, -10.4937) (-1.5743, -11.0619) (-2.0377, -11.3484) (-2.3243, -11.3484) knots 0 0 0 1 2 3 3 3
  spline S26 degree 2 poles (-2.3243, -11.3484) (-2.7903, -11.3484) (-3.0644, -10.9771) knots 0 0 0 1 1 1
  spline S27 degree 2 poles (-3.0644, -10.9771) (-3.2961, -10.6657) (-3.2961, -10.2769) knots 0 0 0 1 1 1
  spline S28 degree 2 poles (-3.2961, -10.2769) (-3.2961, -9.9929) (-3.0145, -9.4322) (-2.556, -9.1656) (-2.2994, -9.1656) knots 0 0 0 1 2 3 3 3
  spline S29 degree 2 poles (-2.3692, -9.3126) (-2.4888, -9.3126) (-2.728, -9.4546) (-2.8775, -9.8085) (-2.8775, -10.0876) knots 0 0 0 1 2 3 3 3
  spline S30 degree 2 poles (-2.8775, -10.0876) (-2.8775, -10.5361) (-2.5212, -11.1889) (-2.2271, -11.1889) knots 0 0 0 1 2 2 2
  spline S31 degree 2 poles (-2.2271, -11.1889) (-2.0103, -11.1889) (-1.7263, -10.8301) (-1.7263, -10.3916) knots 0 0 0 1 2 2 2
  spline S32 degree 2 poles (-1.7263, -10.3916) (-1.7263, -9.8434) (-1.963, -9.5294) knots 0 0 0 1 1 1
  spline S33 degree 2 poles (-1.963, -9.5294) (-2.1225, -9.3126) (-2.3692, -9.3126) knots 0 0 0 1 1 1
  spline S34 degree 2 poles (-0.3881, -9.6066) (-0.1639, -9.3799) (-0.124, -9.345) knots 0 0 0 1 1 1
  spline S35 degree 2 poles (-0.124, -9.345) (-0.0219, -9.2603) (0.2124, -9.1656) (0.327, -9.1656) knots 0 0 0 1 2 2 2
  spline S36 degree 2 poles (0.327, -9.1656) (0.5214, -9.1656) (0.8005, -9.3923) (0.8453, -9.6066) knots 0 0 0 1 2 2 2
  spline S37 degree 2 poles (0.8453, -9.6066) (1.077, -9.335) (1.396, -9.1656) (1.5654, -9.1656) knots 0 0 0 1 2 2 2
  spline S38 degree 2 poles (1.5654, -9.1656) (1.7299, -9.1656) (1.9816, -9.335) (2.0563, -9.5244) knots 0 0 0 1 2 2 2
  spline S39 degree 2 poles (2.0563, -9.5244) (2.1062, -9.6565) (2.1062, -9.9356) knots 0 0 0 1 1 1
  line L28 (2.1062, -9.9356) -> (2.1062, -10.8202)
  spline S40 degree 2 poles (2.1062, -10.8202) (2.1062, -11.012) (2.1361, -11.0843) knots 0 0 0 1 1 1
  spline S41 degree 2 poles (2.1361, -11.0843) (2.1585, -11.1341) (2.2806, -11.2039) (2.4177, -11.2039) knots 0 0 0 1 2 2 2
  line L29 (2.4177, -11.2039) -> (2.4177, -11.2861)
  line L30 (2.4177, -11.2861) -> (1.3985, -11.2861)
  line L31 (1.3985, -11.2861) -> (1.3985, -11.2039)
  line L32 (1.3985, -11.2039) -> (1.4409, -11.2039)
  spline S42 degree 2 poles (1.4409, -11.2039) (1.5754, -11.2039) (1.6502, -11.1516) knots 0 0 0 1 1 1
  spline S43 degree 2 poles (1.6502, -11.1516) (1.7, -11.1167) (1.7224, -11.0369) knots 0 0 0 1 1 1
  spline S44 degree 2 poles (1.7224, -11.0369) (1.7324, -10.9996) (1.7324, -10.8202) knots 0 0 0 1 1 1
  line L33 (1.7324, -10.8202) -> (1.7324, -9.9356)
  spline S45 degree 2 poles (1.7324, -9.9356) (1.7324, -9.6839) (1.6726, -9.5817) knots 0 0 0 1 1 1
  spline S46 degree 2 poles (1.6726, -9.5817) (1.5854, -9.4372) (1.391, -9.4372) knots 0 0 0 1 1 1
  spline S47 degree 2 poles (1.391, -9.4372) (1.2739, -9.4372) (1.0322, -9.5568) (0.8627, -9.7188) knots 0 0 0 1 2 2 2
  line L34 (0.8627, -9.7188) -> (0.8578, -9.7437)
  line L35 (0.8578, -9.7437) -> (0.8627, -9.8384)
  line L36 (0.8627, -9.8384) -> (0.8627, -10.8202)
  spline S48 degree 2 poles (0.8627, -10.8202) (0.8627, -11.032) (0.9101, -11.1341) (1.0397, -11.2039) (1.1967, -11.2039) knots 0 0 0 1 2 3 3 3
  line L37 (1.1967, -11.2039) -> (1.1967, -11.2861)
  line L38 (1.1967, -11.2861) -> (0.1551, -11.2861)
  line L39 (0.1551, -11.2861) -> (0.1551, -11.2039)
  spline S49 degree 2 poles (0.1551, -11.2039) (0.3245, -11.2039) (0.4541, -11.1242) (0.479, -11.0419) knots 0 0 0 1 2 2 2
  spline S50 degree 2 poles (0.479, -11.0419) (0.489, -11.0046) (0.489, -10.8202) knots 0 0 0 1 1 1
  line L40 (0.489, -10.8202) -> (0.489, -9.9356)
  spline S51 degree 2 poles (0.489, -9.9356) (0.489, -9.6839) (0.4142, -9.5742) knots 0 0 0 1 1 1
  spline S52 degree 2 poles (0.4142, -9.5742) (0.317, -9.4297) (0.1401, -9.4297) knots 0 0 0 1 1 1
  spline S53 degree 2 poles (0.1401, -9.4297) (0.018, -9.4297) (-0.1016, -9.4945) knots 0 0 0 1 1 1
  spline S54 degree 2 poles (-0.1016, -9.4945) (-0.286, -9.5942) (-0.3881, -9.7188) knots 0 0 0 1 1 1
  line L41 (-0.3881, -9.7188) -> (-0.3881, -10.8202)
  spline S55 degree 2 poles (-0.3881, -10.8202) (-0.3881, -11.022) (-0.3333, -11.1441) (-0.2212, -11.2039) (-0.0542, -11.2039) knots 0 0 0 1 2 3 3 3
  line L42 (-0.0542, -11.2039) -> (-0.0542, -11.2861)
  line L43 (-0.0542, -11.2861) -> (-1.0759, -11.2861)
  line L44 (-1.0759, -11.2861) -> (-1.0759, -11.2039)
  spline S56 degree 2 poles (-1.0759, -11.2039) (-0.9339, -11.2039) (-0.8217, -11.1441) (-0.7619, -11.012) (-0.7619, -10.8202) knots 0 0 0 1 2 3 3 3
  line L45 (-0.7619, -10.8202) -> (-0.7619, -10.0327)
  spline S57 degree 2 poles (-0.7619, -10.0327) (-0.7619, -9.6939) (-0.7819, -9.5967) knots 0 0 0 1 1 1
  spline S58 degree 2 poles (-0.7819, -9.5967) (-0.7968, -9.5219) (-0.8666, -9.4646) (-0.9239, -9.4646) knots 0 0 0 1 2 2 2
  spline S59 degree 2 poles (-0.9239, -9.4646) (-0.9862, -9.4646) (-1.0734, -9.4995) knots 0 0 0 1 1 1
  line L46 (-1.0734, -9.4995) -> (-1.1083, -9.4173)
  line L47 (-1.1083, -9.4173) -> (-0.4853, -9.1656)
  line L48 (-0.4853, -9.1656) -> (-0.3881, -9.1656)
  line L49 (-0.3881, -9.1656) -> (-0.3881, -9.6066)
  line L50 (5.0067, -11.2039) -> (5.0067, -11.2861)
  line L51 (5.0067, -11.2861) -> (3.7034, -11.2861)
  line L52 (3.7034, -11.2861) -> (3.7034, -11.2039)
  line L53 (3.7034, -11.2039) -> (3.8106, -11.2039)
  spline S60 degree 2 poles (3.8106, -11.2039) (4, -11.2039) (4.0847, -11.0943) knots 0 0 0 1 1 1
  spline S61 degree 2 poles (4.0847, -11.0943) (4.1395, -11.022) (4.1395, -10.7454) knots 0 0 0 1 1 1
  line L54 (4.1395, -10.7454) -> (4.1395, -8.7769)
  spline S62 degree 2 poles (4.1395, -8.7769) (4.1395, -8.5451) (4.1096, -8.4704) knots 0 0 0 1 1 1
  spline S63 degree 2 poles (4.1096, -8.4704) (4.0872, -8.4131) (4.0174, -8.3732) knots 0 0 0 1 1 1
  spline S64 degree 2 poles (4.0174, -8.3732) (3.9202, -8.3184) (3.8106, -8.3184) knots 0 0 0 1 1 1
  line L55 (3.8106, -8.3184) -> (3.7034, -8.3184)
  line L56 (3.7034, -8.3184) -> (3.7034, -8.2361)
  line L57 (3.7034, -8.2361) -> (5.0067, -8.2361)
  line L58 (5.0067, -8.2361) -> (5.0067, -8.3184)
  line L59 (5.0067, -8.3184) -> (4.897, -8.3184)
  spline S65 degree 2 poles (4.897, -8.3184) (4.7126, -8.3184) (4.6254, -8.428) knots 0 0 0 1 1 1
  spline S66 degree 2 poles (4.6254, -8.428) (4.5706, -8.5003) (4.5706, -8.7769) knots 0 0 0 1 1 1
  line L60 (4.5706, -8.7769) -> (4.5706, -10.7454)
  spline S67 degree 2 poles (4.5706, -10.7454) (4.5706, -10.9771) (4.6005, -11.0519) knots 0 0 0 1 1 1
  spline S68 degree 2 poles (4.6005, -11.0519) (4.6229, -11.1092) (4.6927, -11.1491) knots 0 0 0 1 1 1
  spline S69 degree 2 poles (4.6927, -11.1491) (4.7899, -11.2039) (4.897, -11.2039) knots 0 0 0 1 1 1
  line L61 (4.897, -11.2039) -> (5.0067, -11.2039)
  line L62 (6.4993, -9.5942) -> (7.6281, -10.7105)
  spline S70 degree 2 poles (7.6281, -10.7105) (7.9047, -10.9896) (8.2959, -11.1914) (8.4902, -11.2039) knots 0 0 0 1 2 2 2
  line L63 (8.4902, -11.2039) -> (8.4902, -11.2861)
  line L64 (8.4902, -11.2861) -> (7.0375, -11.2861)
  line L65 (7.0375, -11.2861) -> (7.0375, -11.2039)
  spline S71 degree 2 poles (7.0375, -11.2039) (7.1671, -11.2039) (7.2817, -11.1167) (7.2817, -11.0619) knots 0 0 0 1 2 2 2
  spline S72 degree 2 poles (7.2817, -11.0619) (7.2817, -11.007) (7.2393, -10.9223) (7.1197, -10.8052) knots 0 0 0 1 2 2 2
  line L66 (7.1197, -10.8052) -> (6.0682, -9.7636)
  line L67 (6.0682, -9.7636) -> (6.0682, -10.7454)
  spline S73 degree 2 poles (6.0682, -10.7454) (6.0682, -10.9771) (6.0981, -11.0519) knots 0 0 0 1 1 1
  spline S74 degree 2 poles (6.0981, -11.0519) (6.1205, -11.1092) (6.1928, -11.1491) knots 0 0 0 1 1 1
  spline S75 degree 2 poles (6.1928, -11.1491) (6.2875, -11.2039) (6.3971, -11.2039) knots 0 0 0 1 1 1
  line L68 (6.3971, -11.2039) -> (6.4993, -11.2039)
  line L69 (6.4993, -11.2039) -> (6.4993, -11.2861)
  line L70 (6.4993, -11.2861) -> (5.201, -11.2861)
  line L71 (5.201, -11.2861) -> (5.201, -11.2039)
  line L72 (5.201, -11.2039) -> (5.3082, -11.2039)
  spline S76 degree 2 poles (5.3082, -11.2039) (5.4976, -11.2039) (5.5823, -11.0943) knots 0 0 0 1 1 1
  spline S77 degree 2 poles (5.5823, -11.0943) (5.6371, -11.022) (5.6371, -10.7454) knots 0 0 0 1 1 1
  line L73 (5.6371, -10.7454) -> (5.6371, -8.7769)
  spline S78 degree 2 poles (5.6371, -8.7769) (5.6371, -8.5451) (5.6072, -8.4679) knots 0 0 0 1 1 1
  spline S79 degree 2 poles (5.6072, -8.4679) (5.5848, -8.4131) (5.515, -8.3732) knots 0 0 0 1 1 1
  spline S80 degree 2 poles (5.515, -8.3732) (5.4178, -8.3184) (5.3082, -8.3184) knots 0 0 0 1 1 1
  line L74 (5.3082, -8.3184) -> (5.201, -8.3184)
  line L75 (5.201, -8.3184) -> (5.201, -8.2361)
  line L76 (5.201, -8.2361) -> (6.4993, -8.2361)
  line L77 (6.4993, -8.2361) -> (6.4993, -8.3184)
  line L78 (6.4993, -8.3184) -> (6.3971, -8.3184)
  spline S81 degree 2 poles (6.3971, -8.3184) (6.29, -8.3184) (6.1928, -8.3707) knots 0 0 0 1 1 1
  spline S82 degree 2 poles (6.1928, -8.3707) (6.123, -8.4056) (6.0682, -8.5501) (6.0682, -8.7769) knots 0 0 0 1 2 2 2
  line L79 (6.0682, -8.7769) -> (6.0682, -9.7088)
  spline S83 degree 2 poles (6.0682, -9.7088) (6.113, -9.6664) (6.3772, -9.4247) knots 0 0 0 1 1 1
  spline S84 degree 2 poles (6.3772, -9.4247) (7.045, -8.8117) (7.1845, -8.6074) knots 0 0 0 1 1 1
  spline S85 degree 2 poles (7.1845, -8.6074) (7.2443, -8.5152) (7.2443, -8.4479) knots 0 0 0 1 1 1
  spline S86 degree 2 poles (7.2443, -8.4479) (7.2443, -8.3981) (7.1496, -8.3184) (7.0375, -8.3184) knots 0 0 0 1 2 2 2
  line L80 (7.0375, -8.3184) -> (6.9677, -8.3184)
  line L81 (6.9677, -8.3184) -> (6.9677, -8.2361)
  line L82 (6.9677, -8.2361) -> (8.0891, -8.2361)
  line L83 (8.0891, -8.2361) -> (8.0891, -8.3184)
  spline S87 degree 2 poles (8.0891, -8.3184) (7.9919, -8.3209) (7.8274, -8.3707) (7.5957, -8.5127) (7.4237, -8.6697) knots 0 0 0 1 2 3 3 3
  spline S88 degree 2 poles (7.4237, -8.6697) (7.3739, -8.7171) (6.9652, -9.1307) knots 0 0 0 1 1 1
  line L84 (6.9652, -9.1307) -> (6.4993, -9.5942)
  line L85 (9.4122, -8.4031) -> (9.4122, -9.6066)
  line L86 (9.4122, -9.6066) -> (10.0825, -9.6066)
  spline S89 degree 2 poles (10.0825, -9.6066) (10.3442, -9.6066) (10.4314, -9.5269) knots 0 0 0 1 1 1
  spline S90 degree 2 poles (10.4314, -9.5269) (10.551, -9.4247) (10.5634, -9.1631) knots 0 0 0 1 1 1
  line L87 (10.5634, -9.1631) -> (10.6457, -9.1631)
  line L88 (10.6457, -9.1631) -> (10.6457, -10.2271)
  line L89 (10.6457, -10.2271) -> (10.5634, -10.2271)
  spline S91 degree 2 poles (10.5634, -10.2271) (10.5311, -10.0053) (10.5011, -9.943) knots 0 0 0 1 1 1
  spline S92 degree 2 poles (10.5011, -9.943) (10.4588, -9.8633) (10.2744, -9.7736) (10.0825, -9.7736) knots 0 0 0 1 2 2 2
  line L90 (10.0825, -9.7736) -> (9.4122, -9.7736)
  line L91 (9.4122, -9.7736) -> (9.4122, -10.7778)
  spline S93 degree 2 poles (9.4122, -10.7778) (9.4122, -10.9796) (9.4471, -11.0668) (9.5393, -11.1192) (9.6639, -11.1192) knots 0 0 0 1 2 3 3 3
  line L92 (9.6639, -11.1192) -> (10.1822, -11.1192)
  spline S94 degree 2 poles (10.1822, -11.1192) (10.4413, -11.1192) (10.6756, -11.0469) (10.7827, -10.9423) knots 0 0 0 1 2 2 2
  spline S95 degree 2 poles (10.7827, -10.9423) (10.9223, -10.8027) (11.0693, -10.5211) knots 0 0 0 1 1 1
  line L93 (11.0693, -10.5211) -> (11.159, -10.5211)
  line L94 (11.159, -10.5211) -> (10.8949, -11.2861)
  line L95 (10.8949, -11.2861) -> (8.5451, -11.2861)
  line L96 (8.5451, -11.2861) -> (8.5451, -11.2039)
  line L97 (8.5451, -11.2039) -> (8.6522, -11.2039)
  spline S96 degree 2 poles (8.6522, -11.2039) (8.7619, -11.2039) (8.8565, -11.1516) knots 0 0 0 1 1 1
  spline S97 degree 2 poles (8.8565, -11.1516) (8.9288, -11.1142) (8.9811, -10.9697) (8.9811, -10.7454) knots 0 0 0 1 2 2 2
  line L98 (8.9811, -10.7454) -> (8.9811, -8.7669)
  spline S98 degree 2 poles (8.9811, -8.7669) (8.9811, -8.4753) (8.9238, -8.4081) knots 0 0 0 1 1 1
  spline S99 degree 2 poles (8.9238, -8.4081) (8.8416, -8.3184) (8.6522, -8.3184) knots 0 0 0 1 1 1
  line L99 (8.6522, -8.3184) -> (8.5451, -8.3184)
  line L100 (8.5451, -8.3184) -> (8.5451, -8.2361)
  line L101 (8.5451, -8.2361) -> (10.8973, -8.2361)
  line L102 (10.8973, -8.2361) -> (10.9297, -8.9064)
  line L103 (10.9297, -8.9064) -> (10.8425, -8.9064)
  spline S100 degree 2 poles (10.8425, -8.9064) (10.7952, -8.6647) (10.6806, -8.4853) (10.5684, -8.438) knots 0 0 0 1 2 2 2
  spline S101 degree 2 poles (10.5684, -8.438) (10.4787, -8.4031) (10.2495, -8.4031) knots 0 0 0 1 1 1
  line L104 (10.2495, -8.4031) -> (9.4122, -8.4031)
  line L105 (13.3767, -10.267) -> (12.1906, -10.267)
  line L106 (12.1906, -10.267) -> (11.9838, -10.7454)
  spline S102 degree 2 poles (11.9838, -10.7454) (11.9065, -10.9248) (11.9065, -11.012) knots 0 0 0 1 1 1
  spline S103 degree 2 poles (11.9065, -11.012) (11.9065, -11.0818) (12.0411, -11.1889) (12.2604, -11.2039) knots 0 0 0 1 2 2 2
  line L107 (12.2604, -11.2039) -> (12.2604, -11.2861)
  line L108 (12.2604, -11.2861) -> (11.2985, -11.2861)
  line L109 (11.2985, -11.2861) -> (11.2985, -11.2039)
  spline S104 degree 2 poles (11.2985, -11.2039) (11.4904, -11.169) (11.5452, -11.1167) knots 0 0 0 1 1 1
  spline S105 degree 2 poles (11.5452, -11.1167) (11.6598, -11.007) (11.7994, -10.6756) knots 0 0 0 1 1 1
  line L110 (11.7994, -10.6756) -> (12.8759, -8.1664)
  line L111 (12.8759, -8.1664) -> (12.9556, -8.1664)
  line L112 (12.9556, -8.1664) -> (14.0171, -10.703)
  spline S106 degree 2 poles (14.0171, -10.703) (14.1442, -11.0095) (14.3535, -11.1914) (14.5404, -11.2039) knots 0 0 0 1 2 2 2
  line L113 (14.5404, -11.2039) -> (14.5404, -11.2861)
  line L114 (14.5404, -11.2861) -> (13.3369, -11.2861)
  line L115 (13.3369, -11.2861) -> (13.3369, -11.2039)
  spline S107 degree 2 poles (13.3369, -11.2039) (13.5188, -11.1939) (13.6483, -11.0918) (13.6483, -11.017) knots 0 0 0 1 2 2 2
  spline S108 degree 2 poles (13.6483, -11.017) (13.6483, -10.9173) (13.5586, -10.703) knots 0 0 0 1 1 1
  line L116 (13.5586, -10.703) -> (13.3767, -10.267)
  line L117 (13.3069, -10.1) -> (12.7936, -8.8666)
  line L118 (12.7936, -8.8666) -> (12.2629, -10.1)
  line L119 (12.2629, -10.1) -> (13.3069, -10.1)
  spline S109 degree 2 poles (-5.8104, -14.4082) (-5.5114, -13.9896) (-5.1675, -13.9896) knots 0 0 0 1 1 1
  spline S110 degree 2 poles (-5.1675, -13.9896) (-4.851, -13.9896) (-4.3801, -14.5303) (-4.3801, -15.0013) knots 0 0 0 1 2 2 2
  spline S111 degree 2 poles (-4.3801, -15.0013) (-4.3801, -15.5495) (-4.7439, -15.8859) knots 0 0 0 1 1 1